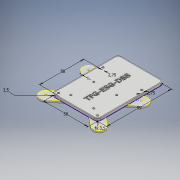
# Autodesk Inventor part: ChasisInferiorDron_SinParedes_P0
Saved by Autodesk Inventor 2017.3 (Build 213256000, 256)
## iProperties
Part Number: ChasisInferiorDron_SinParedes_P0
Material: Genérico
Document SubType Name: Modeling
Designer: danie
Density: 1 g/cm^3
Appearance: Valor por defecto
Author: danie
## iProperties of the stored document ChasisInferiorDron_P0_3DPrint.ipt
Part Number: ChasisInferiorDron_P0_3DPrint
Material: Genérico
Document SubType Name: Modeling
Designer: danie
Density: 1 g/cm^3
Appearance: Valor por defecto
Author: danie
Autodesk Inventor part; units mm, degrees
ref_plane "YZ Plane" through (0, 0, 0) normal (1, 0, 0) x (0, 1, 0)
ref_plane "XZ Plane" through (0, 0, 0) normal (0, 1, 0) x (-1, 0, 0)
ref_plane "XY Plane" through (0, 0, 0) normal (0, 0, 1) x (1, 0, 0)
sketch "Boceto1" plane through (0, 0, 0) normal (0, 0, 1) x (1, 0, 0)
  line L0 (-30.286, -34.1176) -> (39.714, 22.4509)
  line L1 (30.286, 34.1176) -> (-39.714, -22.4509)
  arc A0 (-39.714, -22.4509) -> (-30.286, -34.1176) centre (-35, -28.2843) ccw
  arc A1 (39.714, 22.4509) -> (30.286, 34.1176) centre (35, 28.2843) ccw
  line L2 (-35, 28.2843) -> (35, -28.2843) construction
  line L3 (-39.714, 22.4509) -> (30.286, -34.1176)
  line L4 (39.714, -22.4509) -> (-30.286, 34.1176)
  arc A2 (-30.286, 34.1176) -> (-39.714, 22.4509) centre (-35, 28.2843) ccw
  arc A3 (30.286, -34.1176) -> (39.714, -22.4509) centre (35, -28.2843) ccw
  line L5 (-35, 28.2843) -> (55, 28.2843) construction
  line L6 (-15, -15) -> (-15, 15)
  line L7 (-15, 15) -> (15, 15)
  line L8 (15, 15) -> (15, -15)
  line L9 (15, -15) -> (-15, -15)
  line L10 (-15, -15) -> (15, 15) construction
  line L11 (-15, 15) -> (15, -15) construction
  line L12 (-15, -15) -> (15, -15) construction
  point P0 (-10.2427, 47.1726)
  point P1 (0, 0)
  dimension "d7" = 90
  dimension "d9" = 15
  dimension "d10" = 90
  dimension "d12" = 15
  dimension "d13" = 70
  dimension "d15" = 70
  dimension "d16" = 30
  dimension "d17" = 90
  dimension "d18" = 30
  constraints: 28 end point, 8 point on circle, 8 tangent, 4 centre point, 4 parallel, 3 midpoint, 2 equal length, 2 horizontal, 2 horizontal alignment, 1 perpendicular, 1 vertical
  measures "d7" distance of A0.centre A1.centre
  measures "d9" diameter of A1
  measures "d10" distance of L2.start L2.end
  measures "d12" diameter of A3
  measures "d13" distance of A1.centre L2.start
  measures "d15" distance of L2.end A0.centre
  measures "d16" distance of L6.start L6.end
  measures "d17" angle of L12 L6
  measures "d18" distance of L6.end L7.end
extrude "Extrusión1" add sketch "Boceto1" along normal blind 3
hole "Agujero1" at (35, 28.2843, 3) direction (0, 0, -1) diameter 2.5 end through all
hole "Agujero2" at (35, -28.2843, 3) direction (0, 0, -1) diameter 2.5 end through all
hole "Agujero3" at (-35, -28.2843, 3) direction (0, 0, -1) diameter 2.5 end through all
hole "Agujero4" at (-35, 28.2843, 3) direction (0, 0, -1) diameter 2.5 end through all
hole "Agujero5" at (-15, 15, 3) direction (0, 0, -1) diameter 2.5 end through all
hole "Agujero6" at (-15, -15, 3) direction (0, 0, -1) diameter 2.5 end through all
hole "Agujero7" at (15, -15, 3) direction (0, 0, -1) diameter 2.5 end through all
hole "Agujero8" at (15, 15, 3) direction (0, 0, -1) diameter 2.5 end through all
sketch "Boceto3" plane through (0, 0, 3) normal (0, 0, 1) x (1, 0, 0)
  line L0 (-25.5, 60.8929) -> (25.5, 60.8929)
  line L1 (29, 57.3929) -> (29, -20.6071)
  line L2 (25.5, -24.1071) -> (-25.5, -24.1071)
  line L3 (-29, -20.6071) -> (-29, 57.3929)
  arc A0 (-29, -20.6071) -> (-25.5, -24.1071) centre (-25.5, -20.6071) ccw
  arc A1 (25.5, -24.1071) -> (29, -20.6071) centre (25.5, -20.6071) ccw
  arc A2 (29, 57.3929) -> (25.5, 60.8929) centre (25.5, 57.3929) ccw
  arc A3 (-25.5, 60.8929) -> (-29, 57.3929) centre (-25.5, 57.3929) ccw
  circle A4 centre (15, 15) radius 1.25 projected
  circle A5 centre (15, -15) radius 1.25 projected
  circle A6 centre (-15, -15) radius 1.25 projected
  circle A7 centre (-15, 15) radius 1.25 projected
  circle A8 centre (-35, 28.2843) radius 1.25 projected
  circle A9 centre (-35, -28.2843) radius 1.25 projected
  circle A10 centre (35, -28.2843) radius 1.25 projected
  circle A11 centre (35, 28.2843) radius 1.25 projected
  line L4 (-6.6291, 15) -> (-30.286, 34.1176) projected
  arc A12 (-30.286, 34.1176) -> (-39.714, 22.4509) centre (-35, 28.2843) ccw projected
  line L5 (-39.714, 22.4509) -> (-15, 2.479) projected
  line L6 (-15, 2.479) -> (-15, -2.479) projected
  line L7 (-15, -2.479) -> (-39.714, -22.4509) projected
  arc A13 (-39.714, -22.4509) -> (-30.286, -34.1176) centre (-35, -28.2843) ccw projected
  line L8 (-30.286, -34.1176) -> (-6.6291, -15) projected
  line L9 (-6.6291, -15) -> (6.6291, -15) projected
  line L10 (6.6291, -15) -> (30.286, -34.1176) projected
  arc A14 (30.286, -34.1176) -> (39.714, -22.4509) centre (35, -28.2843) ccw projected
  line L11 (39.714, -22.4509) -> (15, -2.479) projected
  line L12 (15, -2.479) -> (15, 2.479) projected
  line L13 (15, 2.479) -> (39.714, 22.4509) projected
  arc A15 (39.714, 22.4509) -> (30.286, 34.1176) centre (35, 28.2843) ccw projected
  line L14 (30.286, 34.1176) -> (6.6291, 15) projected
  line L15 (6.6291, 15) -> (-6.6291, 15) projected
  line L16 (-35, -28.2843) -> (35, 28.2843) construction
  circle A16 centre (35, -28.2843) radius 1.25 projected
  line L17 (-35, 28.2843) -> (35, -28.2843) construction
  circle A17 centre (-25.5, 37.3929) radius 1.375
  circle A18 centre (25.5, 37.3929) radius 1.375
  line L18 (-4.815, -3.944) -> (-4.815, 39.962) construction
  line L19 (-4.815, 39.962) -> (4.8805, 39.962) construction
  line L20 (4.8805, 39.962) -> (4.8805, -3.944) construction
  line L21 (4.8805, -3.944) -> (-4.815, -3.944) construction
  line L22 (-30, 57.3929) -> (-30, -20.6071)
  arc A19 (-30, -20.6071) -> (-25.5, -25.1071) centre (-25.5, -20.6071) ccw
  line L23 (-25.5, -25.1071) -> (25.5, -25.1071)
  arc A20 (25.5, -25.1071) -> (30, -20.6071) centre (25.5, -20.6071) ccw
  line L24 (30, -20.6071) -> (30, 57.3929)
  arc A21 (30, 57.3929) -> (25.5, 61.8929) centre (25.5, 57.3929) ccw
  line L25 (25.5, 61.8929) -> (-25.5, 61.8929)
  arc A22 (-25.5, 61.8929) -> (-30, 57.3929) centre (-25.5, 57.3929) ccw
  point P0 (0, 0)
  point P1 (29, -24.1071)
  point P2 (29, 60.8929)
  point P3 (-29, -24.1071)
  dimension "d93" = 58
  dimension "d94" = 85
  dimension "d95" = 3.5
  dimension "d96" = 3.5
  dimension "d122" = 2.75
  dimension "d123" = 2.75
  dimension "d124" = 58
  dimension "d195" = 1
  constraints: 20 end point, 16 point on circle, 10 centre point, 9 point on line, 8 tangent, 4 parallel, 2 equal radius, 2 perpendicular, 2 vertical alignment, 1 horizontal, 1 horizontal alignment, 9 other
  measures "d93" distance of point (29, -24.107) point (-29, -24.107)
  measures "d94" distance of point (29, 60.893) point (29, -24.107)
  measures "d95" radius of A0
  measures "d96" radius of A1
  measures "d122" diameter of A17
  measures "d123" diameter of A18
  measures "d124" distance of A0.centre A17.centre
  measures "d195" distance between parallel lines of L3 L22
extrude "Extrusión3" add sketch "Boceto3" along normal blind 3 contours L0 A2 L1 L14 L15 L4 L3 A3 | L4 L15 L14 L1 L13 L12 L11 A1 L2 L10 L9 L8 A0 L3 L7 L6 L5 | L5 L6 L7 L3 | L1 L11 L12 L13 | L8 L9 L10 L2
hole "Agujero11" at (-25.5, -20.6071, 6) direction (0, 0, -1) diameter 2.75 end through all
hole "Agujero12" at (25.5, -20.6071, 6) direction (0, 0, -1) diameter 2.75 end through all
sketch "Boceto4" plane through (0, 0, 6) normal (0, 0, 1) x (1, 0, 0)
  line L0 (-3.4142, -10.4693) -> (-3.4142, 46.7293) construction
  line L1 (-3.4142, 46.7293) -> (2.9329, 46.7293) construction
  line L2 (2.9329, 46.7293) -> (2.9329, -10.4693) construction
  line L3 (2.9329, -10.4693) -> (-3.4142, -10.4693) construction
  line L4 (2.8044, -8.665) -> (-2.1339, -8.665)
  line L5 (-2.1339, -8.665) -> (-2.1339, -10.4693)
  line L6 (-2.1339, -10.4693) -> (-3.2956, -10.4693)
  line L7 (-3.2956, -10.4693) -> (-3.2956, -5.3283)
  line L8 (-3.2956, -5.3283) -> (-2.1339, -5.3283)
  line L9 (-2.1339, -5.3283) -> (-2.1339, -7.1326)
  line L10 (-2.1339, -7.1326) -> (2.8044, -7.1326)
  line L11 (2.8044, -7.1326) -> (2.8044, -8.665)
  line L12 (-2.1339, -0.6173) -> (-2.1339, -3.1779)
  line L13 (-2.1339, -3.1779) -> (-0.9822, -3.1779)
  line L14 (-0.9822, -3.1779) -> (-0.9822, -0.82)
  line L15 (-0.9822, -0.82) -> (0.1795, -0.82)
  line L16 (0.1795, -0.82) -> (0.1795, -3.1779)
  line L17 (0.1795, -3.1779) -> (2.8044, -3.1779)
  line L18 (2.8044, -3.1779) -> (2.8044, -4.7005)
  line L19 (2.8044, -4.7005) -> (-3.2956, -4.7005)
  line L20 (-3.2956, -4.7005) -> (-3.2956, -0.6173)
  line L21 (-3.2956, -0.6173) -> (-2.1339, -0.6173)
  spline S0 degree 2 poles (2.4584, 5.2652) (2.6215, 4.8648) (2.9329, 3.5845) (2.9329, 2.9616) knots 0 0 0 1 2 2 2
  spline S1 degree 2 poles (2.9329, 2.9616) (2.9329, 1.5231) (1.272, -0.1823) (-0.2506, -0.1823) knots 0 0 0 1 2 2 2
  spline S2 degree 2 poles (-0.2506, -0.1823) (-1.6841, -0.1823) (-3.4142, 1.5231) (-3.4142, 3.0061) knots 0 0 0 1 2 2 2
  spline S3 degree 2 poles (-3.4142, 3.0061) (-3.4142, 3.7723) (-3.1226, 4.7313) (-2.8754, 5.2404) knots 0 0 0 1 2 2 2
  line L22 (-2.8754, 5.2404) -> (-1.4419, 5.2404)
  line L23 (-1.4419, 5.2404) -> (-1.4419, 5.102)
  spline S4 degree 2 poles (-1.4419, 5.102) (-1.5259, 4.9933) (-1.8472, 4.578) (-1.956, 4.3803) knots 0 0 0 1 2 2 2
  spline S5 degree 2 poles (-1.956, 4.3803) (-2.0894, 4.1529) (-2.2773, 3.5498) (-2.2773, 3.2137) knots 0 0 0 1 2 2 2
  spline S6 degree 2 poles (-2.2773, 3.2137) (-2.2773, 2.8232) (-2.0301, 2.1756) (-1.778, 1.9235) knots 0 0 0 1 2 2 2
  spline S7 degree 2 poles (-1.778, 1.9235) (-1.5309, 1.6813) (-0.7745, 1.3995) (-0.2753, 1.3995) knots 0 0 0 1 2 2 2
  spline S8 degree 2 poles (-0.2753, 1.3995) (0.7925, 1.3995) (1.8108, 2.4722) (1.8108, 3.3966) knots 0 0 0 1 2 2 2
  spline S9 degree 2 poles (1.8108, 3.3966) (1.8108, 3.4806) (1.8009, 3.6981) (1.796, 3.7822) knots 0 0 0 1 2 2 2
  line L24 (1.796, 3.7822) -> (0.5947, 3.7822)
  line L25 (0.5947, 3.7822) -> (0.5947, 2.6007)
  line L26 (0.5947, 2.6007) -> (-0.5471, 2.6007)
  line L27 (-0.5471, 2.6007) -> (-0.5471, 5.2652)
  line L28 (-0.5471, 5.2652) -> (2.4584, 5.2652)
  line L29 (0.6788, 8.9528) -> (0.6788, 6.239)
  line L30 (0.6788, 6.239) -> (-0.4582, 6.239)
  line L31 (-0.4582, 6.239) -> (-0.4582, 8.9528)
  line L32 (-0.4582, 8.9528) -> (0.6788, 8.9528)
  line L33 (2.8044, 10.0404) -> (-3.2956, 10.0404)
  line L34 (-3.2956, 10.0404) -> (-3.2956, 14.1631)
  line L35 (-3.2956, 14.1631) -> (-2.1339, 14.1631)
  line L36 (-2.1339, 14.1631) -> (-2.1339, 11.5629)
  line L37 (-2.1339, 11.5629) -> (-1.0612, 11.5629)
  line L38 (-1.0612, 11.5629) -> (-1.0612, 13.9604)
  line L39 (-1.0612, 13.9604) -> (0.1004, 13.9604)
  line L40 (0.1004, 13.9604) -> (0.1004, 11.5629)
  line L41 (0.1004, 11.5629) -> (1.6427, 11.5629)
  line L42 (1.6427, 11.5629) -> (1.6427, 14.1631)
  line L43 (1.6427, 14.1631) -> (2.8044, 14.1631)
  line L44 (2.8044, 14.1631) -> (2.8044, 10.0404)
  spline S10 degree 2 poles (2.9131, 17.0845) (2.9131, 16.3826) (2.6413, 15.3247) (2.4435, 14.8699) knots 0 0 0 1 2 2 2
  line L45 (2.4435, 14.8699) -> (0.9902, 14.8699)
  line L46 (0.9902, 14.8699) -> (0.9902, 15.0084)
  spline S11 degree 2 poles (0.9902, 15.0084) (1.3807, 15.4681) (1.8009, 16.5704) (1.8009, 17.0895) knots 0 0 0 1 2 2 2
  spline S12 degree 2 poles (1.8009, 17.0895) (1.8009, 17.2229) (1.7416, 17.653) (1.6823, 17.7815) knots 0 0 0 1 2 2 2
  spline S13 degree 2 poles (1.6823, 17.7815) (1.6131, 17.9397) (1.361, 18.1622) (1.1583, 18.1622) knots 0 0 0 1 2 2 2
  spline S14 degree 2 poles (1.1583, 18.1622) (0.9259, 18.1622) (0.6392, 17.8013) (0.575, 17.5541) knots 0 0 0 1 2 2 2
  spline S15 degree 2 poles (0.575, 17.5541) (0.4909, 17.2427) (0.3476, 16.5358) (0.2388, 16.2244) knots 0 0 0 1 2 2 2
  spline S16 degree 2 poles (0.2388, 16.2244) (-0.0083, 15.5175) (-0.8536, 14.9045) (-1.4864, 14.9045) knots 0 0 0 1 2 2 2
  spline S17 degree 2 poles (-1.4864, 14.9045) (-2.3416, 14.9045) (-3.4044, 16.3529) (-3.4044, 17.4404) knots 0 0 0 1 2 2 2
  spline S18 degree 2 poles (-3.4044, 17.4404) (-3.4044, 17.9842) (-3.1819, 19.0618) (-2.9941, 19.487) knots 0 0 0 1 2 2 2
  line L47 (-2.9941, 19.487) -> (-1.6001, 19.487)
  line L48 (-1.6001, 19.487) -> (-1.6001, 19.3535)
  spline S19 degree 2 poles (-1.6001, 19.3535) (-1.8917, 19.0124) (-2.2921, 18.0336) (-2.2921, 17.5195) knots 0 0 0 1 2 2 2
  spline S20 degree 2 poles (-2.2921, 17.5195) (-2.2921, 17.3169) (-2.2328, 17.0005) (-2.1537, 16.8225) knots 0 0 0 1 2 2 2
  spline S21 degree 2 poles (-2.1537, 16.8225) (-2.0894, 16.6792) (-1.8324, 16.4716) (-1.6742, 16.4716) knots 0 0 0 1 2 2 2
  spline S22 degree 2 poles (-1.6742, 16.4716) (-1.4369, 16.4716) (-1.1651, 16.8028) (-1.0563, 17.2773) knots 0 0 0 1 2 2 2
  spline S23 degree 2 poles (-1.0563, 17.2773) (-0.9871, 17.5838) (-0.8536, 18.1523) (-0.7399, 18.4785) knots 0 0 0 1 2 2 2
  spline S24 degree 2 poles (-0.7399, 18.4785) (-0.5076, 19.1113) (0.2635, 19.7292) (0.8963, 19.7292) knots 0 0 0 1 2 2 2
  spline S25 degree 2 poles (0.8963, 19.7292) (1.8059, 19.7292) (2.9131, 18.3006) (2.9131, 17.0845) knots 0 0 0 1 2 2 2
  spline S26 degree 2 poles (2.4584, 25.6067) (2.6215, 25.2063) (2.9329, 23.926) (2.9329, 23.3032) knots 0 0 0 1 2 2 2
  spline S27 degree 2 poles (2.9329, 23.3032) (2.9329, 21.8647) (1.272, 20.1592) (-0.2506, 20.1592) knots 0 0 0 1 2 2 2
  spline S28 degree 2 poles (-0.2506, 20.1592) (-1.6841, 20.1592) (-3.4142, 21.8647) (-3.4142, 23.3477) knots 0 0 0 1 2 2 2
  spline S29 degree 2 poles (-3.4142, 23.3477) (-3.4142, 24.1139) (-3.1226, 25.0729) (-2.8754, 25.582) knots 0 0 0 1 2 2 2
  line L49 (-2.8754, 25.582) -> (-1.4419, 25.582)
  line L50 (-1.4419, 25.582) -> (-1.4419, 25.4436)
  spline S30 degree 2 poles (-1.4419, 25.4436) (-1.5259, 25.3349) (-1.8472, 24.9196) (-1.956, 24.7219) knots 0 0 0 1 2 2 2
  spline S31 degree 2 poles (-1.956, 24.7219) (-2.0894, 24.4945) (-2.2773, 23.8914) (-2.2773, 23.5553) knots 0 0 0 1 2 2 2
  spline S32 degree 2 poles (-2.2773, 23.5553) (-2.2773, 23.1648) (-2.0301, 22.5172) (-1.778, 22.2651) knots 0 0 0 1 2 2 2
  spline S33 degree 2 poles (-1.778, 22.2651) (-1.5309, 22.0229) (-0.7745, 21.7411) (-0.2753, 21.7411) knots 0 0 0 1 2 2 2
  spline S34 degree 2 poles (-0.2753, 21.7411) (0.7925, 21.7411) (1.8108, 22.8138) (1.8108, 23.7382) knots 0 0 0 1 2 2 2
  spline S35 degree 2 poles (1.8108, 23.7382) (1.8108, 23.8222) (1.8009, 24.0397) (1.796, 24.1238) knots 0 0 0 1 2 2 2
  line L51 (1.796, 24.1238) -> (0.5947, 24.1238)
  line L52 (0.5947, 24.1238) -> (0.5947, 22.9423)
  line L53 (0.5947, 22.9423) -> (-0.5471, 22.9423)
  line L54 (-0.5471, 22.9423) -> (-0.5471, 25.6067)
  line L55 (-0.5471, 25.6067) -> (2.4584, 25.6067)
  line L56 (0.6788, 29.2944) -> (0.6788, 26.5806)
  line L57 (0.6788, 26.5806) -> (-0.4582, 26.5806)
  line L58 (-0.4582, 26.5806) -> (-0.4582, 29.2944)
  line L59 (-0.4582, 29.2944) -> (0.6788, 29.2944)
  spline S36 degree 2 poles (-0.2407, 35.8245) (0.6145, 35.8245) (1.9591, 35.078) (2.32, 34.5096) knots 0 0 0 1 2 2 2
  spline S37 degree 2 poles (2.32, 34.5096) (2.6264, 34.035) (2.8044, 32.9178) (2.8044, 32.29) knots 0 0 0 1 2 2 2
  line L60 (2.8044, 32.29) -> (2.8044, 30.3819)
  line L61 (2.8044, 30.3819) -> (-3.2956, 30.3819)
  line L62 (-3.2956, 30.3819) -> (-3.2956, 32.2703)
  spline S38 degree 2 poles (-3.2956, 32.2703) (-3.2956, 32.9129) (-3.1325, 34.035) (-2.8161, 34.5293) knots 0 0 0 1 2 2 2
  spline S39 degree 2 poles (-2.8161, 34.5293) (-2.4305, 35.1275) (-1.1255, 35.8245) (-0.2407, 35.8245) knots 0 0 0 1 2 2 2
  spline S40 degree 2 poles (-0.2506, 34.2525) (-0.8536, 34.2525) (-1.7138, 33.8373) (-1.956, 33.4122) knots 0 0 0 1 2 2 2
  spline S41 degree 2 poles (-1.956, 33.4122) (-2.1241, 33.1007) (-2.1587, 32.4186) (-2.1587, 31.944) knots 0 0 0 1 2 2 2
  line L63 (-2.1587, 31.944) -> (-2.1587, 31.9144)
  line L64 (-2.1587, 31.9144) -> (1.6625, 31.9144)
  line L65 (1.6625, 31.9144) -> (1.6625, 31.944)
  spline S42 degree 2 poles (1.6625, 31.944) (1.6625, 32.4581) (1.6279, 33.165) (1.4252, 33.4863) knots 0 0 0 1 2 2 2
  spline S43 degree 2 poles (1.4252, 33.4863) (1.1879, 33.862) (0.3525, 34.2525) (-0.2506, 34.2525) knots 0 0 0 1 2 2 2
  spline S44 degree 2 poles (2.9131, 38.6174) (2.9131, 37.9155) (2.6413, 36.8576) (2.4435, 36.4028) knots 0 0 0 1 2 2 2
  line L66 (2.4435, 36.4028) -> (0.9902, 36.4028)
  line L67 (0.9902, 36.4028) -> (0.9902, 36.5413)
  spline S45 degree 2 poles (0.9902, 36.5413) (1.3807, 37.001) (1.8009, 38.1033) (1.8009, 38.6224) knots 0 0 0 1 2 2 2
  spline S46 degree 2 poles (1.8009, 38.6224) (1.8009, 38.7558) (1.7416, 39.1859) (1.6823, 39.3144) knots 0 0 0 1 2 2 2
  spline S47 degree 2 poles (1.6823, 39.3144) (1.6131, 39.4726) (1.361, 39.6951) (1.1583, 39.6951) knots 0 0 0 1 2 2 2
  spline S48 degree 2 poles (1.1583, 39.6951) (0.9259, 39.6951) (0.6392, 39.3342) (0.575, 39.087) knots 0 0 0 1 2 2 2
  spline S49 degree 2 poles (0.575, 39.087) (0.4909, 38.7756) (0.3476, 38.0687) (0.2388, 37.7573) knots 0 0 0 1 2 2 2
  spline S50 degree 2 poles (0.2388, 37.7573) (-0.0083, 37.0504) (-0.8536, 36.4374) (-1.4864, 36.4374) knots 0 0 0 1 2 2 2
  spline S51 degree 2 poles (-1.4864, 36.4374) (-2.3416, 36.4374) (-3.4044, 37.8858) (-3.4044, 38.9733) knots 0 0 0 1 2 2 2
  spline S52 degree 2 poles (-3.4044, 38.9733) (-3.4044, 39.5171) (-3.1819, 40.5947) (-2.9941, 41.0199) knots 0 0 0 1 2 2 2
  line L68 (-2.9941, 41.0199) -> (-1.6001, 41.0199)
  line L69 (-1.6001, 41.0199) -> (-1.6001, 40.8864)
  spline S53 degree 2 poles (-1.6001, 40.8864) (-1.8917, 40.5453) (-2.2921, 39.5665) (-2.2921, 39.0524) knots 0 0 0 1 2 2 2
  spline S54 degree 2 poles (-2.2921, 39.0524) (-2.2921, 38.8498) (-2.2328, 38.5334) (-2.1537, 38.3554) knots 0 0 0 1 2 2 2
  spline S55 degree 2 poles (-2.1537, 38.3554) (-2.0894, 38.2121) (-1.8324, 38.0045) (-1.6742, 38.0045) knots 0 0 0 1 2 2 2
  spline S56 degree 2 poles (-1.6742, 38.0045) (-1.4369, 38.0045) (-1.1651, 38.3357) (-1.0563, 38.8102) knots 0 0 0 1 2 2 2
  spline S57 degree 2 poles (-1.0563, 38.8102) (-0.9871, 39.1167) (-0.8536, 39.6852) (-0.7399, 40.0114) knots 0 0 0 1 2 2 2
  spline S58 degree 2 poles (-0.7399, 40.0114) (-0.5076, 40.6442) (0.2635, 41.2621) (0.8963, 41.2621) knots 0 0 0 1 2 2 2
  spline S59 degree 2 poles (0.8963, 41.2621) (1.8059, 41.2621) (2.9131, 39.8335) (2.9131, 38.6174) knots 0 0 0 1 2 2 2
  spline S60 degree 2 poles (2.9131, 43.9315) (2.9131, 43.2295) (2.6413, 42.1716) (2.4435, 41.7169) knots 0 0 0 1 2 2 2
  line L70 (2.4435, 41.7169) -> (0.9902, 41.7169)
  line L71 (0.9902, 41.7169) -> (0.9902, 41.8553)
  spline S61 degree 2 poles (0.9902, 41.8553) (1.3807, 42.315) (1.8009, 43.4174) (1.8009, 43.9364) knots 0 0 0 1 2 2 2
  spline S62 degree 2 poles (1.8009, 43.9364) (1.8009, 44.0699) (1.7416, 44.4999) (1.6823, 44.6285) knots 0 0 0 1 2 2 2
  spline S63 degree 2 poles (1.6823, 44.6285) (1.6131, 44.7866) (1.361, 45.0091) (1.1583, 45.0091) knots 0 0 0 1 2 2 2
  spline S64 degree 2 poles (1.1583, 45.0091) (0.9259, 45.0091) (0.6392, 44.6482) (0.575, 44.4011) knots 0 0 0 1 2 2 2
  spline S65 degree 2 poles (0.575, 44.4011) (0.4909, 44.0896) (0.3476, 43.3827) (0.2388, 43.0713) knots 0 0 0 1 2 2 2
  spline S66 degree 2 poles (0.2388, 43.0713) (-0.0083, 42.3644) (-0.8536, 41.7515) (-1.4864, 41.7515) knots 0 0 0 1 2 2 2
  spline S67 degree 2 poles (-1.4864, 41.7515) (-2.3416, 41.7515) (-3.4044, 43.1998) (-3.4044, 44.2874) knots 0 0 0 1 2 2 2
  spline S68 degree 2 poles (-3.4044, 44.2874) (-3.4044, 44.8311) (-3.1819, 45.9088) (-2.9941, 46.3339) knots 0 0 0 1 2 2 2
  line L72 (-2.9941, 46.3339) -> (-1.6001, 46.3339)
  line L73 (-1.6001, 46.3339) -> (-1.6001, 46.2004)
  spline S69 degree 2 poles (-1.6001, 46.2004) (-1.8917, 45.8593) (-2.2921, 44.8806) (-2.2921, 44.3665) knots 0 0 0 1 2 2 2
  spline S70 degree 2 poles (-2.2921, 44.3665) (-2.2921, 44.1638) (-2.2328, 43.8474) (-2.1537, 43.6695) knots 0 0 0 1 2 2 2
  spline S71 degree 2 poles (-2.1537, 43.6695) (-2.0894, 43.5261) (-1.8324, 43.3185) (-1.6742, 43.3185) knots 0 0 0 1 2 2 2
  spline S72 degree 2 poles (-1.6742, 43.3185) (-1.4369, 43.3185) (-1.1651, 43.6497) (-1.0563, 44.1242) knots 0 0 0 1 2 2 2
  spline S73 degree 2 poles (-1.0563, 44.1242) (-0.9871, 44.4307) (-0.8536, 44.9992) (-0.7399, 45.3255) knots 0 0 0 1 2 2 2
  spline S74 degree 2 poles (-0.7399, 45.3255) (-0.5076, 45.9582) (0.2635, 46.5761) (0.8963, 46.5761) knots 0 0 0 1 2 2 2
  spline S75 degree 2 poles (0.8963, 46.5761) (1.8059, 46.5761) (2.9131, 45.1475) (2.9131, 43.9315) knots 0 0 0 1 2 2 2
  point P0 (0, 0)
  constraints: 2 other
extrude "Extrusión4" cut sketch "Boceto4" against normal blind 1
extrude "Extrusión7" add sketch "Boceto3" along normal up to surface (3 mm away) separate body contours A3 L3 L4 L22 A22 L25 A21 L24 L14 L1 A2 L0 | L3 L5 L22 L4 | L14 L24 L13 L1 | L3 L7 L22 L5 | L13 L24 L11 L1 | L3 A0 L2 L8 L23 A19 L22 L7 | L11 L24 A20 L23 L10 L2 A1 L1 | L2 L10 L23 L8
equation "\"d96\" = d95"
